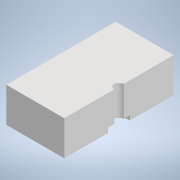
# Autodesk Inventor part: 15_Base_Dietro
Saved by Autodesk Inventor 2020 (Build 240168000, 168)
## iProperties
Created: 2019-10-17
Part Number: 15_Base_Dietro
Material: Generico
Document SubType Name: Modeling
Designer: socci
Density: 1 g/cm^3
Appearance: Default
Author: socci
Autodesk Inventor part; units mm, degrees
ref_plane "YZ Plane" through (0, 0, 0) normal (1, 0, 0) x (0, 1, 0)
ref_plane "XZ Plane" through (0, 0, 0) normal (0, 1, 0) x (-1, 0, 0)
ref_plane "XY Plane" through (0, 0, 0) normal (0, 0, 1) x (1, 0, 0)
sketch "Schizzo1" plane through (0, 0, 0) normal (0, 1, 0) x (-1, 0, 0)
  line L0 (25, 47.2222) -> (-25, 47.2222)
  line L1 (-25, 47.2222) -> (-25, -47.2222)
  line L2 (-25, -47.2222) -> (25, -47.2222)
  line L3 (25, -47.2222) -> (25, 47.2222)
  line L4 (25, 47.2222) -> (-25, -47.2222) construction
  line L5 (-25, 47.2222) -> (25, -47.2222) construction
  point P0 (0, 0)
  point P1 (0, 0)
  point P2 (0, 0)
  dimension "d0" = 50
  constraints: 12 end point, 3 midpoint, 2 parallel, 1 coincident, 1 horizontal, 1 perpendicular
  measures "d0" distance of L0.start L0.end
extrude "Estrusione1" add sketch "Schizzo1" along normal blind 16
sketch "Schizzo2" plane through (0, 0, 0) normal (0, -1, 0) x (1, 0, 0)
  circle A0 centre (25, 0) radius 9.5
  line L0 (25, 47.2222) -> (25, -47.2222) projected
  point P0 (0, 0)
  dimension "d3" = 19
  constraints: 1 centre point, 1 coincident, 1 midpoint
  measures "d3" diameter of A0
extrude "Estrusione2" cut sketch "Schizzo2" against normal blind 4
sketch "Schizzo4" plane through (0, 4, 0) normal (0, -1, 0) x (1, 0, 0)
  circle A0 centre (25, 0) radius 6
  line L0 (25, 9.5) -> (25, -9.5) projected
  point P0 (0, 0)
  point P1 (25, 6)
  point P2 (25, -6)
  dimension "d6" = 12
  constraints: 1 centre point, 1 coincident, 1 midpoint
  measures "d6" diameter of A0
extrude "Estrusione3" cut sketch "Schizzo4" against normal blind 26 contours L0 A0 picked at (23.13, -0.7092)
